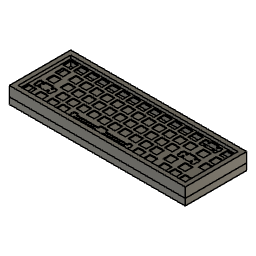
Case(in progress) v1 (Autodesk Fusion 360 design; units mm, degrees)
Autodesk Fusion 360 part; units mm, degrees
sketch "Sketch1" plane through (0, 0, 0) normal (0, 0, 1) x (1, 0, 0)
  line L0 (0.0951, 95.5075) -> (304.895, 95.5075)
  line L1 (304.895, 95.5075) -> (304.895, 0.2577)
  line L2 (304.895, 0.2577) -> (0.0951, 0.2577)
  line L3 (0.0951, 0.2577) -> (0.0951, 95.5075)
  line L4 (133.587, 16.7831) -> (133.587, 12.0826)
  line L5 (133.587, 12.0826) -> (93.9631, 12.0826)
  line L6 (93.9631, 12.0826) -> (93.9631, 15.3128)
  line L7 (93.9631, 15.3128) -> (87.212, 15.3128)
  line L8 (87.212, 15.3128) -> (87.212, 12.0826)
  line L9 (87.212, 12.0826) -> (86.3879, 12.0826)
  line L10 (86.3879, 12.0826) -> (86.3879, 9.2838)
  line L11 (86.3879, 9.2838) -> (87.212, 9.2838)
  line L12 (87.212, 9.2838) -> (87.212, 3.0138)
  line L13 (87.212, 3.0138) -> (88.937, 3.0138)
  line L14 (88.937, 3.0138) -> (88.937, 1.8135)
  line L15 (88.937, 1.8135) -> (92.2376, 1.8135)
  line L16 (92.2376, 1.8135) -> (92.2376, 3.0138)
  line L17 (92.2376, 3.0138) -> (93.9631, 3.0138)
  line L18 (93.9631, 3.0138) -> (93.9631, 7.4841)
  line L19 (93.9631, 7.4841) -> (133.587, 7.4841)
  line L20 (133.587, 7.4841) -> (133.587, 2.7836)
  line L21 (133.587, 2.7836) -> (147.588, 2.7836)
  line L22 (147.588, 2.7836) -> (147.588, 7.4841)
  line L23 (147.588, 7.4841) -> (187.212, 7.4841)
  line L24 (187.212, 7.4841) -> (187.212, 3.0138)
  line L25 (187.212, 3.0138) -> (188.937, 3.0138)
  line L26 (188.937, 3.0138) -> (188.937, 1.8135)
  line L27 (188.937, 1.8135) -> (192.238, 1.8135)
  line L28 (192.238, 1.8135) -> (192.238, 3.0138)
  line L29 (192.238, 3.0138) -> (193.963, 3.0138)
  line L30 (193.963, 3.0138) -> (193.963, 9.2838)
  line L31 (193.963, 9.2838) -> (194.787, 9.2838)
  line L32 (194.787, 9.2838) -> (194.787, 12.0826)
  line L33 (194.787, 12.0826) -> (193.963, 12.0826)
  line L34 (193.963, 12.0826) -> (193.963, 15.3128)
  line L35 (193.963, 15.3128) -> (187.212, 15.3128)
  line L36 (187.212, 15.3128) -> (187.212, 12.0826)
  line L37 (187.212, 12.0826) -> (147.588, 12.0826)
  line L38 (147.588, 12.0826) -> (147.588, 16.7831)
  line L39 (147.588, 16.7831) -> (133.587, 16.7831)
  line L40 (2.6197, 16.7831) -> (16.6192, 16.7831)
  line L41 (16.6192, 16.7831) -> (16.6192, 2.7836)
  line L42 (16.6192, 2.7836) -> (2.6196, 2.7836)
  line L43 (2.6197, 2.7836) -> (2.6197, 16.7831)
  line L44 (24.0509, 16.7831) -> (38.0503, 16.7831)
  line L45 (38.0503, 16.7831) -> (38.0503, 2.7836)
  line L46 (38.0503, 2.7836) -> (24.0509, 2.7836)
  line L47 (24.0509, 2.7836) -> (24.0509, 16.7831)
  line L48 (45.4822, 16.7831) -> (59.4815, 16.7831)
  line L49 (59.4815, 16.7831) -> (59.4815, 2.7836)
  line L50 (59.4815, 2.7836) -> (45.4822, 2.7836)
  line L51 (45.4822, 2.7836) -> (45.4822, 16.7831)
  line L52 (64.5322, 16.7831) -> (78.5315, 16.7831)
  line L53 (78.5315, 16.7831) -> (78.5315, 2.7836)
  line L54 (78.5315, 2.7836) -> (64.5322, 2.7836)
  line L55 (64.5322, 2.7836) -> (64.5322, 16.7831)
  line L56 (202.645, 16.7831) -> (216.644, 16.7831)
  line L57 (216.644, 16.7831) -> (216.644, 2.7836)
  line L58 (216.644, 2.7836) -> (202.645, 2.7836)
  line L59 (202.645, 2.7836) -> (202.645, 16.7831)
  line L60 (224.076, 16.7831) -> (238.075, 16.7831)
  line L61 (238.075, 16.7831) -> (238.075, 2.7836)
  line L62 (238.075, 2.7836) -> (224.076, 2.7836)
  line L63 (224.076, 2.7836) -> (224.076, 16.7831)
  line L64 (250.27, 16.7831) -> (264.269, 16.7831)
  line L65 (264.269, 16.7831) -> (264.269, 2.7836)
  line L66 (264.269, 2.7836) -> (250.27, 2.7836)
  line L67 (250.27, 2.7836) -> (250.27, 16.7831)
  line L68 (269.32, 16.7831) -> (283.319, 16.7831)
  line L69 (283.319, 16.7831) -> (283.319, 2.7836)
  line L70 (283.319, 2.7836) -> (269.32, 2.7836)
  line L71 (269.32, 2.7836) -> (269.32, 16.7831)
  line L72 (288.37, 16.7831) -> (302.369, 16.7831)
  line L73 (302.369, 16.7831) -> (302.369, 2.7836)
  line L74 (302.369, 2.7836) -> (288.37, 2.7836)
  line L75 (288.37, 2.7836) -> (288.37, 16.7831)
  line L76 (14.5259, 35.833) -> (14.5259, 31.1326)
  line L77 (14.5259, 31.1326) -> (13.0004, 31.1326)
  line L78 (13.0004, 31.1326) -> (13.0004, 34.3628)
  line L79 (13.0004, 34.3628) -> (6.2508, 34.3628)
  line L80 (6.2508, 34.3628) -> (6.2508, 31.1326)
  line L81 (6.2508, 31.1326) -> (5.4253, 31.1326)
  line L82 (5.4253, 31.1326) -> (5.4253, 28.3338)
  line L83 (5.4253, 28.3338) -> (6.2508, 28.3338)
  line L84 (6.2508, 28.3338) -> (6.2508, 22.0638)
  line L85 (6.2508, 22.0638) -> (7.9761, 22.0638)
  line L86 (7.9761, 22.0638) -> (7.9761, 20.8635)
  line L87 (7.9761, 20.8635) -> (11.2751, 20.8635)
  line L88 (11.2751, 20.8635) -> (11.2751, 22.0638)
  line L89 (11.2751, 22.0638) -> (13.0004, 22.0638)
  line L90 (13.0004, 22.0638) -> (13.0004, 26.5327)
  line L91 (13.0004, 26.5327) -> (14.5259, 26.5327)
  line L92 (14.5259, 26.5327) -> (14.5259, 21.8336)
  line L93 (14.5259, 21.8336) -> (28.5254, 21.8336)
  line L94 (28.5254, 21.8336) -> (28.5254, 26.5327)
  line L95 (28.5254, 26.5327) -> (30.0509, 26.5327)
  line L96 (30.0509, 26.5327) -> (30.0509, 22.0638)
  line L97 (30.0509, 22.0638) -> (31.7748, 22.0638)
  line L98 (31.7748, 22.0638) -> (31.7748, 20.8635)
  line L99 (31.7748, 20.8635) -> (35.0752, 20.8635)
  line L100 (35.0752, 20.8635) -> (35.0752, 22.0638)
  line L101 (35.0752, 22.0638) -> (36.8004, 22.0638)
  line L102 (36.8004, 22.0638) -> (36.8004, 28.3338)
  line L103 (36.8004, 28.3338) -> (37.6259, 28.3338)
  line L104 (37.6259, 28.3338) -> (37.6259, 31.1326)
  line L105 (37.6259, 31.1326) -> (36.8004, 31.1326)
  line L106 (36.8004, 31.1326) -> (36.8004, 34.3628)
  line L107 (36.8004, 34.3628) -> (30.0509, 34.3628)
  line L108 (30.0509, 34.3628) -> (30.0509, 31.1326)
  line L109 (30.0509, 31.1326) -> (28.5254, 31.1326)
  line L110 (28.5254, 31.1326) -> (28.5254, 35.833)
  line L111 (28.5254, 35.833) -> (14.5259, 35.833)
  line L112 (45.4822, 35.833) -> (59.4815, 35.833)
  line L113 (59.4815, 35.833) -> (59.4815, 21.8336)
  line L114 (59.4815, 21.8336) -> (45.4822, 21.8336)
  line L115 (45.4822, 21.8336) -> (45.4822, 35.833)
  line L116 (64.5322, 35.833) -> (78.5315, 35.833)
  line L117 (78.5315, 35.833) -> (78.5315, 21.8336)
  line L118 (78.5315, 21.8336) -> (64.5322, 21.8336)
  line L119 (64.5322, 21.8336) -> (64.5322, 35.833)
  line L120 (83.5822, 35.833) -> (97.5815, 35.833)
  line L121 (97.5815, 35.833) -> (97.5815, 21.8336)
  line L122 (97.5815, 21.8336) -> (83.5822, 21.8336)
  line L123 (83.5822, 21.8336) -> (83.5822, 35.833)
  line L124 (102.632, 35.833) -> (116.632, 35.833)
  line L125 (116.632, 35.833) -> (116.632, 21.8336)
  line L126 (116.632, 21.8336) -> (102.632, 21.8336)
  line L127 (102.632, 21.8336) -> (102.632, 35.833)
  line L128 (121.682, 35.833) -> (135.682, 35.833)
  line L129 (135.682, 35.833) -> (135.682, 21.8336)
  line L130 (135.682, 21.8336) -> (121.682, 21.8336)
  line L131 (121.682, 21.8336) -> (121.682, 35.833)
  line L132 (140.732, 35.833) -> (154.732, 35.833)
  line L133 (154.732, 35.833) -> (154.732, 21.8336)
  line L134 (154.732, 21.8336) -> (140.732, 21.8336)
  line L135 (140.732, 21.8336) -> (140.732, 35.833)
  line L136 (159.782, 35.833) -> (173.782, 35.833)
  line L137 (173.782, 35.833) -> (173.782, 21.8336)
  line L138 (173.782, 21.8336) -> (159.782, 21.8336)
  line L139 (159.782, 21.8336) -> (159.782, 35.833)
  line L140 (178.832, 35.833) -> (192.832, 35.833)
  line L141 (192.832, 35.833) -> (192.832, 21.8336)
  line L142 (192.832, 21.8336) -> (178.832, 21.8336)
  line L143 (178.832, 21.8336) -> (178.832, 35.833)
  line L144 (197.882, 35.833) -> (211.882, 35.833)
  line L145 (211.882, 35.833) -> (211.882, 21.8336)
  line L146 (211.882, 21.8336) -> (197.882, 21.8336)
  line L147 (197.882, 21.8336) -> (197.882, 35.833)
  line L148 (216.932, 35.833) -> (230.932, 35.833)
  line L149 (230.932, 35.833) -> (230.932, 21.8336)
  line L150 (230.932, 21.8336) -> (216.932, 21.8336)
  line L151 (216.932, 21.8336) -> (216.932, 35.833)
  line L152 (243.126, 35.833) -> (257.125, 35.833)
  line L153 (257.125, 35.833) -> (257.125, 21.8336)
  line L154 (257.125, 21.8336) -> (243.126, 21.8336)
  line L155 (243.126, 21.8336) -> (243.126, 35.833)
  line L156 (269.32, 35.833) -> (283.319, 35.833)
  line L157 (283.319, 35.833) -> (283.319, 21.8336)
  line L158 (283.319, 21.8336) -> (269.32, 21.8336)
  line L159 (269.32, 21.8336) -> (269.32, 35.833)
  line L160 (257.412, 54.8831) -> (257.412, 50.1826)
  line L161 (257.412, 50.1826) -> (255.888, 50.1826)
  line L162 (255.888, 50.1826) -> (255.888, 53.4127)
  line L163 (255.888, 53.4127) -> (249.137, 53.4127)
  line L164 (249.137, 53.4127) -> (249.137, 50.1826)
  line L165 (249.137, 50.1826) -> (248.313, 50.1826)
  line L166 (248.313, 50.1826) -> (248.313, 47.3837)
  line L167 (248.313, 47.3837) -> (249.137, 47.3837)
  line L168 (249.137, 47.3837) -> (249.137, 41.1138)
  line L169 (249.137, 41.1138) -> (250.862, 41.1138)
  line L170 (250.862, 41.1138) -> (250.862, 39.9136)
  line L171 (250.862, 39.9136) -> (254.161, 39.9136)
  line L172 (254.161, 39.9136) -> (254.161, 41.1138)
  line L173 (254.161, 41.1138) -> (255.888, 41.1138)
  line L174 (255.888, 41.1138) -> (255.888, 45.5828)
  line L175 (255.888, 45.5828) -> (257.412, 45.5828)
  line L176 (257.412, 45.5828) -> (257.412, 40.8838)
  line L177 (257.412, 40.8838) -> (271.413, 40.8838)
  line L178 (271.413, 40.8838) -> (271.413, 45.5828)
  line L179 (271.413, 45.5828) -> (272.937, 45.5828)
  line L180 (272.937, 45.5828) -> (272.937, 41.1138)
  line L181 (272.937, 41.1138) -> (274.662, 41.1138)
  line L182 (274.662, 41.1138) -> (274.662, 39.9136)
  line L183 (274.662, 39.9136) -> (277.963, 39.9136)
  line L184 (277.963, 39.9136) -> (277.963, 41.1138)
  line L185 (277.963, 41.1138) -> (279.688, 41.1138)
  line L186 (279.688, 41.1138) -> (279.688, 47.3837)
  line L187 (279.688, 47.3837) -> (280.512, 47.3837)
  line L188 (280.512, 47.3837) -> (280.512, 50.1826)
  line L189 (280.512, 50.1826) -> (279.688, 50.1826)
  line L190 (279.688, 50.1826) -> (279.688, 53.4127)
  line L191 (279.688, 53.4127) -> (272.937, 53.4127)
  line L192 (272.937, 53.4127) -> (272.937, 50.1826)
  line L193 (272.937, 50.1826) -> (271.413, 50.1826)
  line L194 (271.413, 50.1826) -> (271.413, 54.8831)
  line L195 (271.413, 54.8831) -> (257.412, 54.8831)
  line L196 (9.762, 54.8831) -> (23.7629, 54.8831)
  line L197 (23.7629, 54.8831) -> (23.7629, 40.8838)
  line L198 (23.7629, 40.8838) -> (9.762, 40.8838)
  line L199 (9.762, 40.8838) -> (9.762, 54.8831)
  line L200 (35.9572, 54.8831) -> (49.9565, 54.8831)
  line L201 (49.9565, 54.8831) -> (49.9565, 40.8838)
  line L202 (49.9565, 40.8838) -> (35.9572, 40.8838)
  line L203 (35.9572, 40.8838) -> (35.9572, 54.8831)
  line L204 (55.0072, 54.8831) -> (69.0065, 54.8831)
  line L205 (69.0065, 54.8831) -> (69.0065, 40.8838)
  line L206 (69.0065, 40.8838) -> (55.0072, 40.8838)
  line L207 (55.0072, 40.8838) -> (55.0072, 54.8831)
  line L208 (74.0572, 54.8831) -> (88.0565, 54.8831)
  line L209 (88.0565, 54.8831) -> (88.0565, 40.8838)
  line L210 (88.0565, 40.8838) -> (74.0572, 40.8838)
  line L211 (74.0572, 40.8838) -> (74.0572, 54.8831)
  line L212 (93.1072, 54.8831) -> (107.107, 54.8831)
  line L213 (107.107, 54.8831) -> (107.107, 40.8838)
  line L214 (107.107, 40.8838) -> (93.1072, 40.8838)
  line L215 (93.1072, 40.8838) -> (93.1072, 54.8831)
  line L216 (112.157, 54.8831) -> (126.157, 54.8831)
  line L217 (126.157, 54.8831) -> (126.157, 40.8838)
  line L218 (126.157, 40.8838) -> (112.157, 40.8838)
  line L219 (112.157, 40.8838) -> (112.157, 54.8831)
  line L220 (131.207, 54.8831) -> (145.207, 54.8831)
  line L221 (145.207, 54.8831) -> (145.207, 40.8838)
  line L222 (145.207, 40.8838) -> (131.207, 40.8838)
  line L223 (131.207, 40.8838) -> (131.207, 54.8831)
  line L224 (150.257, 54.8831) -> (164.257, 54.8831)
  line L225 (164.257, 54.8831) -> (164.257, 40.8838)
  line L226 (164.257, 40.8838) -> (150.257, 40.8838)
  line L227 (150.257, 40.8838) -> (150.257, 54.8831)
  line L228 (169.307, 54.8831) -> (183.307, 54.8831)
  line L229 (183.307, 54.8831) -> (183.307, 40.8838)
  line L230 (183.307, 40.8838) -> (169.307, 40.8838)
  line L231 (169.307, 40.8838) -> (169.307, 54.8831)
  line L232 (188.357, 54.8831) -> (202.357, 54.8831)
  line L233 (202.357, 54.8831) -> (202.357, 40.8838)
  line L234 (202.357, 40.8838) -> (188.357, 40.8838)
  line L235 (188.357, 40.8838) -> (188.357, 54.8831)
  line L236 (207.407, 54.8831) -> (221.407, 54.8831)
  line L237 (221.407, 54.8831) -> (221.407, 40.8838)
  line L238 (221.407, 40.8838) -> (207.407, 40.8838)
  line L239 (207.407, 40.8838) -> (207.407, 54.8831)
  line L240 (226.457, 54.8831) -> (240.457, 54.8831)
  line L241 (240.457, 54.8831) -> (240.457, 40.8838)
  line L242 (240.457, 40.8838) -> (226.457, 40.8838)
  line L243 (226.457, 40.8838) -> (226.457, 54.8831)
  line L244 (288.37, 54.8831) -> (302.369, 54.8831)
  line L245 (302.369, 54.8831) -> (302.369, 40.8838)
  line L246 (302.369, 40.8838) -> (288.37, 40.8838)
  line L247 (288.37, 40.8838) -> (288.37, 54.8831)
  line L248 (7.3822, 73.9331) -> (21.3817, 73.9331)
  line L249 (21.3817, 73.9331) -> (21.3817, 59.9338)
  line L250 (21.3817, 59.9338) -> (7.3822, 59.9338)
  line L251 (7.3822, 59.9338) -> (7.3822, 73.9331)
  line L252 (31.1947, 73.9331) -> (45.194, 73.9331)
  line L253 (45.194, 73.9331) -> (45.194, 59.9338)
  line L254 (45.194, 59.9338) -> (31.1947, 59.9338)
  line L255 (31.1947, 59.9338) -> (31.1947, 73.9331)
  line L256 (50.2447, 73.9331) -> (64.244, 73.9331)
  line L257 (64.244, 73.9331) -> (64.244, 59.9338)
  line L258 (64.244, 59.9338) -> (50.2447, 59.9338)
  line L259 (50.2447, 59.9338) -> (50.2447, 73.9331)
  line L260 (69.2947, 73.9331) -> (83.294, 73.9331)
  line L261 (83.294, 73.9331) -> (83.294, 59.9338)
  line L262 (83.294, 59.9338) -> (69.2947, 59.9338)
  line L263 (69.2947, 59.9338) -> (69.2947, 73.9331)
  line L264 (88.3447, 73.9331) -> (102.344, 73.9331)
  line L265 (102.344, 73.9331) -> (102.344, 59.9338)
  line L266 (102.344, 59.9338) -> (88.3447, 59.9338)
  line L267 (88.3447, 59.9338) -> (88.3447, 73.9331)
  line L268 (107.395, 73.9331) -> (121.394, 73.9331)
  line L269 (121.394, 73.9331) -> (121.394, 59.9338)
  line L270 (121.394, 59.9338) -> (107.395, 59.9338)
  line L271 (107.395, 59.9338) -> (107.395, 73.9331)
  line L272 (126.445, 73.9331) -> (140.444, 73.9331)
  line L273 (140.444, 73.9331) -> (140.444, 59.9338)
  line L274 (140.444, 59.9338) -> (126.445, 59.9338)
  line L275 (126.445, 59.9338) -> (126.445, 73.9331)
  line L276 (145.495, 73.9331) -> (159.494, 73.9331)
  line L277 (159.494, 73.9331) -> (159.494, 59.9338)
  line L278 (159.494, 59.9338) -> (145.495, 59.9338)
  line L279 (145.495, 59.9338) -> (145.495, 73.9331)
  line L280 (164.545, 73.9331) -> (178.544, 73.9331)
  line L281 (178.544, 73.9331) -> (178.544, 59.9338)
  line L282 (178.544, 59.9338) -> (164.545, 59.9338)
  line L283 (164.545, 59.9338) -> (164.545, 73.9331)
  line L284 (183.595, 73.9331) -> (197.594, 73.9331)
  line L285 (197.594, 73.9331) -> (197.594, 59.9338)
  line L286 (197.594, 59.9338) -> (183.595, 59.9338)
  line L287 (183.595, 59.9338) -> (183.595, 73.9331)
  line L288 (202.645, 73.9331) -> (216.644, 73.9331)
  line L289 (216.644, 73.9331) -> (216.644, 59.9338)
  line L290 (216.644, 59.9338) -> (202.645, 59.9338)
  line L291 (202.645, 59.9338) -> (202.645, 73.9331)
  line L292 (221.695, 73.9331) -> (235.694, 73.9331)
  line L293 (235.694, 73.9331) -> (235.694, 59.9338)
  line L294 (235.694, 59.9338) -> (221.695, 59.9338)
  line L295 (221.695, 59.9338) -> (221.695, 73.9331)
  line L296 (240.745, 73.9331) -> (254.744, 73.9331)
  line L297 (254.744, 73.9331) -> (254.744, 59.9338)
  line L298 (254.744, 59.9338) -> (240.745, 59.9338)
  line L299 (240.745, 59.9338) -> (240.745, 73.9331)
  line L300 (264.557, 73.9331) -> (278.557, 73.9331)
  line L301 (278.557, 73.9331) -> (278.557, 59.9338)
  line L302 (278.557, 59.9338) -> (264.557, 59.9338)
  line L303 (264.557, 59.9338) -> (264.557, 73.9331)
  line L304 (288.37, 73.9331) -> (302.369, 73.9331)
  line L305 (302.369, 73.9331) -> (302.369, 59.9338)
  line L306 (302.369, 59.9338) -> (288.37, 59.9338)
  line L307 (288.37, 59.9338) -> (288.37, 73.9331)
  line L308 (259.795, 92.9831) -> (259.795, 88.2826)
  line L309 (259.795, 88.2826) -> (258.269, 88.2826)
  line L310 (258.269, 88.2826) -> (258.269, 91.5127)
  line L311 (258.269, 91.5127) -> (251.52, 91.5127)
  line L312 (251.52, 91.5127) -> (251.52, 88.2826)
  line L313 (251.52, 88.2826) -> (250.694, 88.2826)
  line L314 (250.694, 88.2826) -> (250.694, 85.4837)
  line L315 (250.694, 85.4837) -> (251.52, 85.4837)
  line L316 (251.52, 85.4837) -> (251.52, 79.2138)
  line L317 (251.52, 79.2138) -> (253.243, 79.2138)
  line L318 (253.243, 79.2138) -> (253.243, 78.0136)
  line L319 (253.243, 78.0136) -> (256.544, 78.0136)
  line L320 (256.544, 78.0136) -> (256.544, 79.2138)
  line L321 (256.544, 79.2138) -> (258.269, 79.2138)
  line L322 (258.269, 79.2138) -> (258.269, 83.6828)
  line L323 (258.269, 83.6828) -> (259.795, 83.6828)
  line L324 (259.795, 83.6828) -> (259.795, 78.9838)
  line L325 (259.795, 78.9838) -> (273.794, 78.9838)
  line L326 (273.794, 78.9838) -> (273.794, 83.6828)
  line L327 (273.794, 83.6828) -> (275.32, 83.6828)
  line L328 (275.32, 83.6828) -> (275.32, 79.2138)
  line L329 (275.32, 79.2138) -> (277.045, 79.2138)
  line L330 (277.045, 79.2138) -> (277.045, 78.0136)
  line L331 (277.045, 78.0136) -> (280.344, 78.0136)
  line L332 (280.344, 78.0136) -> (280.344, 79.2138)
  line L333 (280.344, 79.2138) -> (282.069, 79.2138)
  line L334 (282.069, 79.2138) -> (282.069, 85.4837)
  line L335 (282.069, 85.4837) -> (282.895, 85.4837)
  line L336 (282.895, 85.4837) -> (282.895, 88.2826)
  line L337 (282.895, 88.2826) -> (282.069, 88.2826)
  line L338 (282.069, 88.2826) -> (282.069, 91.5127)
  line L339 (282.069, 91.5127) -> (275.32, 91.5127)
  line L340 (275.32, 91.5127) -> (275.32, 88.2826)
  line L341 (275.32, 88.2826) -> (273.794, 88.2826)
  line L342 (273.794, 88.2826) -> (273.794, 92.9831)
  line L343 (273.794, 92.9831) -> (259.795, 92.9831)
  line L344 (2.6197, 92.9831) -> (16.6192, 92.9831)
  line L345 (16.6192, 92.9831) -> (16.6192, 78.9838)
  line L346 (16.6192, 78.9838) -> (2.6196, 78.9838)
  line L347 (2.6197, 78.9838) -> (2.6197, 92.9831)
  line L348 (21.6697, 92.9831) -> (35.669, 92.9831)
  line L349 (35.669, 92.9831) -> (35.669, 78.9838)
  line L350 (35.669, 78.9838) -> (21.6697, 78.9838)
  line L351 (21.6697, 78.9838) -> (21.6697, 92.9831)
  line L352 (40.7197, 92.9831) -> (54.719, 92.9831)
  line L353 (54.719, 92.9831) -> (54.719, 78.9838)
  line L354 (54.719, 78.9838) -> (40.7197, 78.9838)
  line L355 (40.7197, 78.9838) -> (40.7197, 92.9831)
  line L356 (59.7697, 92.9831) -> (73.769, 92.9831)
  line L357 (73.769, 92.9831) -> (73.769, 78.9838)
  line L358 (73.769, 78.9838) -> (59.7697, 78.9838)
  line L359 (59.7697, 78.9838) -> (59.7697, 92.9831)
  line L360 (78.8197, 92.9831) -> (92.819, 92.9831)
  line L361 (92.819, 92.9831) -> (92.819, 78.9838)
  line L362 (92.819, 78.9838) -> (78.8197, 78.9838)
  line L363 (78.8197, 78.9838) -> (78.8197, 92.9831)
  line L364 (97.8683, 92.9831) -> (111.869, 92.9831)
  line L365 (111.869, 92.9831) -> (111.869, 78.9838)
  line L366 (111.869, 78.9838) -> (97.8683, 78.9838)
  line L367 (97.8683, 78.9838) -> (97.8683, 92.9831)
  line L368 (116.918, 92.9831) -> (130.919, 92.9831)
  line L369 (130.919, 92.9831) -> (130.919, 78.9838)
  line L370 (130.919, 78.9838) -> (116.918, 78.9838)
  line L371 (116.918, 78.9838) -> (116.918, 92.9831)
  line L372 (135.97, 92.9831) -> (149.969, 92.9831)
  line L373 (149.969, 92.9831) -> (149.969, 78.9838)
  line L374 (149.969, 78.9838) -> (135.97, 78.9838)
  line L375 (135.97, 78.9838) -> (135.97, 92.9831)
  line L376 (155.02, 92.9831) -> (169.019, 92.9831)
  line L377 (169.019, 92.9831) -> (169.019, 78.9838)
  line L378 (169.019, 78.9838) -> (155.02, 78.9838)
  line L379 (155.02, 78.9838) -> (155.02, 92.9831)
  line L380 (174.07, 92.9831) -> (188.069, 92.9831)
  line L381 (188.069, 92.9831) -> (188.069, 78.9838)
  line L382 (188.069, 78.9838) -> (174.07, 78.9838)
  line L383 (174.07, 78.9838) -> (174.07, 92.9831)
  line L384 (193.12, 92.9831) -> (207.119, 92.9831)
  line L385 (207.119, 92.9831) -> (207.119, 78.9838)
  line L386 (207.119, 78.9838) -> (193.12, 78.9838)
  line L387 (193.12, 78.9838) -> (193.12, 92.9831)
  line L388 (212.17, 92.9831) -> (226.169, 92.9831)
  line L389 (226.169, 92.9831) -> (226.169, 78.9838)
  line L390 (226.169, 78.9838) -> (212.17, 78.9838)
  line L391 (212.17, 78.9838) -> (212.17, 92.9831)
  line L392 (231.22, 92.9831) -> (245.219, 92.9831)
  line L393 (245.219, 92.9831) -> (245.219, 78.9838)
  line L394 (245.219, 78.9838) -> (231.22, 78.9838)
  line L395 (231.22, 78.9838) -> (231.22, 92.9831)
  line L396 (288.37, 92.9831) -> (302.369, 92.9831)
  line L397 (302.369, 92.9831) -> (302.369, 78.9838)
  line L398 (302.369, 78.9838) -> (288.37, 78.9838)
  line L399 (288.37, 78.9838) -> (288.37, 92.9831)
  line L400 (305.395, -0.2423) -> (-0.4049, -0.2423)
  line L401 (-0.4049, -0.2423) -> (-0.4049, 96.0075)
  line L402 (-0.4049, 96.0075) -> (305.395, 96.0075)
  line L403 (305.395, 96.0075) -> (305.395, -0.2423)
  line L404 (313.395, -8.2423) -> (-8.4049, -8.2423)
  line L405 (-8.4049, -8.2423) -> (-8.4049, 104.0075)
  line L406 (-8.4049, 104.0075) -> (313.395, 104.0075)
  line L407 (313.395, 104.0075) -> (313.395, -8.2423)
  dimension "d1" = -0.5
  dimension "d2" = -8.5
extrude "Extrude1" add sketch "Sketch1" along normal blind 1.5 contours L0 L1 L2 L3 makes body 1
extrude "Extrude2" add sketch "Sketch1" along normal blind 18 separate body contours L404 L405 L406 L407 makes body 2
extrude "Extrude3" add sketch "Sketch1" against normal blind 12 separate body contours L0 L1 L2 L3 | L4 L5 L6 L7 L8 L9 L10 L11 L12 L13 L14 L15 L16 L17 L18 L19 L20 L21 L22 L23 L24 L25 L26 L27 L28 L29 L30 L31 L32 L33 L34 L35 L36 L37 L38 L39 | L40 L41 L42 L43 | L44 L45 L46 L47 | L48 L49 L50 L51 | L52 L53 L54 L55 | L56 L57 L58 L59 | L60 L61 L62 L63 | L64 L65 L66 L67 | L68 L69 L70 L71 | L72 L73 L74 L75 | L76 L77 L78 L79 L80 L81 L82 L83 L84 L85 L86 L87 L88 L89 L90 L91 L92 L93 L94 L95 L96 L97 L98 L99 L100 L101 L102 L103 L104 L105 L106 L107 L108 L109 L110 L111 | L112 L113 L114 L115 | L116 L117 L118 L119 | L120 L121 L122 L123 | L124 L125 L126 L127 | L128 L129 L130 L131 | L132 L133 L134 L135 | L136 L137 L138 L139 | L140 L141 L142 L143 | L144 L145 L146 L147 | L148 L149 L150 L151 | L152 L153 L154 L155 | L156 L157 L158 L159 | L160 L161 L162 L163 L164 L165 L166 L167 L168 L169 L170 L171 L172 L173 L174 L175 L176 L177 L178 L179 L180 L181 L182 L183 L184 L185 L186 L187 L188 L189 L190 L191 L192 L193 L194 L195 | L196 L197 L198 L199 | L200 L201 L202 L203 | L204 L205 L206 L207 | L208 L209 L210 L211 | L212 L213 L214 L215 | L216 L217 L218 L219 | L220 L221 L222 L223 | L224 L225 L226 L227 | L228 L229 L230 L231 | L232 L233 L234 L235 | L236 L237 L238 L239 | L240 L241 L242 L243 | L244 L245 L246 L247 | L248 L249 L250 L251 | L252 L253 L254 L255 | L256 L257 L258 L259 | L260 L261 L262 L263 | L264 L265 L266 L267 | L268 L269 L270 L271 | L272 L273 L274 L275 | L276 L277 L278 L279 | L280 L281 L282 L283 | L284 L285 L286 L287 | L288 L289 L290 L291 | L292 L293 L294 L295 | L296 L297 L298 L299 | L300 L301 L302 L303 | L304 L305 L306 L307 | L308 L309 L310 L311 L312 L313 L314 L315 L316 L317 L318 L319 L320 L321 L322 L323 L324 L325 L326 L327 L328 L329 L330 L331 L332 L333 L334 L335 L336 L337 L338 L339 L340 L341 L342 L343 | L344 L345 L346 L347 | L348 L349 L350 L351 | L352 L353 L354 L355 | L356 L357 L358 L359 | L360 L361 L362 L363 | L364 L365 L366 L367 | L368 L369 L370 L371 | L372 L373 L374 L375 | L376 L377 L378 L379 | L380 L381 L382 L383 | L384 L385 L386 L387 | L388 L389 L390 L391 | L392 L393 L394 L395 | L396 L397 L398 L399 | L400 L401 L402 L403 | L404 L405 L406 L407 makes body 3
move_body "Move1" bodies 1 to x (1, 0, 0) y (0, 1, 0) z (0, 0, 1) at (0, 0, 11.1)
named bodies: "plate"
